Autodesk Fusion 360 part; units mm, degrees
(part 2 of 2)
sketch "Skizze5" plane through (0, 0, 6) normal (0, 0, 1) x (1, 0, 0)
  line L0 (-42, 58.3839) -> (-42, -1.6351) construction
  line L1 (-53.2037, 40.24) -> (-25.198, 40.24) construction
  line L2 (-52.8872, 9.76) -> (-24.0904, 9.76) construction
  line L3 (-69.9754, 25) -> (-16.6539, 25) construction
  line L4 (-40.2968, 37.29) -> (-38.5936, 40.24)
  line L5 (-38.5936, 40.24) -> (-40.2968, 43.19)
  line L6 (-40.2968, 43.19) -> (-43.7032, 43.19)
  line L7 (-43.7032, 43.19) -> (-45.4064, 40.24)
  line L8 (-45.4064, 40.24) -> (-43.7032, 37.29)
  line L9 (-43.7032, 37.29) -> (-40.2968, 37.29)
  line L10 (-40.2968, 6.81) -> (-38.5936, 9.76)
  line L11 (-38.5936, 9.76) -> (-40.2968, 12.71)
  line L12 (-40.2968, 12.71) -> (-43.7032, 12.71)
  line L13 (-43.7032, 12.71) -> (-45.4064, 9.76)
  line L14 (-45.4064, 9.76) -> (-43.7032, 6.81)
  line L15 (-43.7032, 6.81) -> (-40.2968, 6.81)
  line L16 (-28, 68.4623) -> (-28, -7.051) construction
  line L17 (-20.4, 58.9387) -> (-20.4, 26.026) construction
  line L18 (7.5, 60.7966) -> (7.5, 32.5289) construction
  line L19 (-25.5, 3.9958) -> (-25.5, -8.4792) construction
  line L20 (22.7, 6.3547) -> (22.7, -11) construction
  line L21 (16.5548, -1.7) -> (36, -1.7) construction
  line L22 (-31, 49.1) -> (26, 49.1) construction
  line L23 (-35.2993, -3) -> (-15, -3) construction
  point P0 (-42, 40.24)
  point P1 (-42, 9.76)
  point P2 (-42, 40.24)
  point P3 (-42, 9.76)
  point P4 (-25.5, -3)
  point P5 (22.7, -1.7)
  point P6 (-20.4, 49.1)
  dimension "d197" = 42
  dimension "d198" = 25
  dimension "d199" = 15.24
  dimension "d200" = 15.24
  dimension "d201" = 5.9
  dimension "d202" = 5.9
  dimension "d343" = 28
  dimension "d344" = 7.6
  dimension "d345" = 27.9
  dimension "d346" = 2.5
  dimension "d347" = 48.2
  dimension "d349" = 49.1
  dimension "d350" = 50.8
  dimension "d351" = 1.3
  constraint vertical L0
  constraint horizontal L1
  constraint horizontal L2
  constraint horizontal L3
  constraint coincident L1 P2
  constraint coincident L0 P2
  constraint coincident L2 P3
  constraint coincident L0 P3
  constraint coincident P2 P0
  constraint coincident P3 P1
  constraint vertical L16
  constraint perpendicular L3 L17
  constraint vertical L18
  constraint vertical L19
  constraint perpendicular L1 L20
  constraint perpendicular L20 L21
  constraint perpendicular L16 L22
  constraint perpendicular L16 L23
  constraint coincident L23 P4
  constraint coincident L19 P4
  constraint coincident L21 P5
  constraint coincident L20 P5
  constraint coincident L17 P6
  constraint coincident L22 P6
  measures "d197" distance of L0 origin
  measures "d198" distance of L3 origin
  measures "d199" distance of L1 L3
  measures "d200" distance of L2 L3
  measures "d201" distance of L6 L9
  measures "d202" distance of L12 L15
  measures "d343" distance of origin L16
  measures "d344" distance of L16 L17
  measures "d345" distance of L17 L18
  measures "d346" distance of L16 L19
  measures "d347" distance of L19 L20
  measures "d349" distance of origin L22
  measures "d350" distance of L21 L22
  measures "d351" distance of L21 L23
extrude "Extrusion12" cut sketch "Skizze5" along normal blind 2.6 bodies 11
sketch "Skizze6" plane through (0, 0, 10.3) normal (0, 0, 1) x (-1, 0, 0)
  circle A0 centre (42, -9.76) radius 4
  line L0 (93.3037, -25) -> (4.6405, -25) construction
  line L1 (42, -47.4403) -> (42, 6.0922) construction
  line L2 (54.3254, -40.24) -> (21.704, -40.24) construction
  line L3 (59.0095, -9.76) -> (18.86, -9.76) construction
  line L4 (33, -49.1) -> (-20.9546, -49.1) construction
  line L5 (33, 3) -> (13, 3) construction
  line L6 (-12.3565, 1.7) -> (-33, 1.7) construction
  line L7 (28, -59.161) -> (28, -2) construction
  line L8 (20.4, -59) -> (20.4, -30.5278) construction
  line L9 (25.5, -4.5907) -> (25.5, 13) construction
  line L10 (-22.7, -6.3058) -> (-22.7, 11) construction
  line L11 (-7.5, -59) -> (-7.5, -40) construction
  point P0 (42, -40.24)
  point P1 (42, -9.76)
  point P2 (20.4, -49.1)
  point P3 (25.5, 3)
  point P4 (20.4, -49.1)
  point P5 (-22.7, 1.7)
  dimension "d205" = 25
  dimension "d206" = 42
  dimension "d207" = 15.24
  dimension "d208" = 15.24
  dimension "d352" = 49.1
  dimension "d353" = 50.8
  dimension "d354" = 1.3
  dimension "d355" = 28
  dimension "d356" = 7.6
  dimension "d357" = 2.5
  dimension "d358" = 48.2
  dimension "d359" = 27.9
  constraint horizontal L0
  constraint vertical L1
  constraint horizontal L2
  constraint horizontal L3
  constraint coincident L2 P0
  constraint coincident L1 P0
  constraint coincident A0.centre P1
  constraint horizontal L4
  constraint horizontal L5
  constraint horizontal L6
  constraint perpendicular L4 L7
  constraint vertical L8
  constraint vertical L9
  constraint parallel L1 L10
  constraint vertical L11
  constraint coincident L5 P3
  constraint coincident L9 P3
  constraint coincident P4 P2
  constraint coincident L10 P5
  constraint coincident L6 P5
  measures "d205" distance of L0 origin
  measures "d206" distance of origin L1
  measures "d207" distance of L0 L2
  measures "d208" distance of L0 L3
  measures "d352" distance of L4 origin
  measures "d353" distance of L4 L6
  measures "d354" distance of L5 L6
  measures "d355" distance of origin L7
  measures "d356" distance of L7 L8
  measures "d357" distance of L7 L9
  measures "d358" distance of L9 L10
  measures "d359" distance of L11 P4
hole "Bohrung6" at (-42, 40.24, 10.3) at (-42, 9.76, 10.3) direction (0, 0, -1) diameter 3.5 depth 8.5 tip angle 180 bodies 11
extrude "Extrusion13" add sketch "Skizze1" along normal blind 2 separate body contours A41 makes body 27
extrude "Extrusion14" add sketch "Skizze1" along normal blind 3 contours A43 A50 | A43 A50 bodies 11
extrude "Extrusion15" add sketch "Skizze1" along normal blind 22.9 separate body contours L69 A55 | L36 L69 L95 A55 A56 makes body 28
extrude "Extrusion23" add sketch "Skizze1" along normal blind 10.3 contours L36 L69 L99 L103 A52 A53 | L69 L103 A52 | A57 L106 | A58 picked at (-22.0084, 48.4127) picked at (22.7471, -2.8734) bodies 11
sketch "Skizze7" plane through (0, 0, 22.9) normal (0, 0, 1) x (-1, 0, 0)
  arc A0 (-4.3775, -51.6) -> (-10.6225, -51.6) centre (-7.5, -49.1) ccw
  line L0 (-10.6225, -51.6) -> (-4.3775, -51.6)
  line L1 (20.4, -59.2047) -> (20.4, -39) construction
  line L2 (28, -63.0503) -> (28, 11) construction
  line L3 (25.5, -8) -> (25.5, 11) construction
  line L4 (-7.5, -58) -> (-7.5, -40) construction
  line L5 (-22.7, -5) -> (-22.7, 13) construction
  line L6 (33, -49.1) -> (-18.5705, -49.1) construction
  line L7 (-16.5833, 1.7) -> (-30, 1.7) construction
  line L8 (34, 3) -> (-38, 3) construction
  point P0 (20.4, -49.1024)
  point P1 (-7.5, -49.1)
  point P2 (-22.7, 1.7)
  point P3 (25.5, 3)
  dimension "d251" = 28
  dimension "d252" = 7.6
  dimension "d253" = 2.5
  dimension "d254" = 27.9
  dimension "d255" = 48.2
  dimension "d257" = 49.1
  dimension "d258" = 50.8
  dimension "d259" = 1.3
  constraint vertical L1
  constraint vertical L2
  constraint vertical L3
  constraint vertical L4
  constraint parallel L2 L5
  constraint perpendicular L4 L6
  constraint horizontal L7
  constraint perpendicular L2 L8
  constraint midpoint L1 P0
  constraint coincident P1 A0.centre
  constraint coincident L5 P2
  constraint coincident L7 P2
  constraint coincident L8 P3
  constraint coincident L3 P3
  measures "d251" distance of origin L2
  measures "d252" distance of L1 L2
  measures "d253" distance of L2 L3
  measures "d254" distance of L1 L4
  measures "d255" distance of L3 L5
  measures "d257" distance of origin L6
  measures "d258" distance of L6 L7
  measures "d259" distance of L7 L8
hole "Bohrung7" at (7.5, 49.1, 22.9) direction (0, 0, -1) diameter 2.4 depth 20 tip angle 180 bodies 11 28
hole "Bohrung11" at (-20.4, 49.1, 10.3) at (-25.5, -3, 10.3) at (22.7, -1.7, 10.3) direction (0, 0, -1) diameter 2.4 depth 8 tip angle 180 bodies 11
ref_plane "Arbeitsebene3" through (0, 0, 18.5) normal (0, 0, 1) x (1, 0, 0)
sketch "Skizze8" plane through (0, 0, 18.5) normal (0, 0, 1) x (1, 0, 0)
  line L0 (-32.3311, 49.1) -> (45.7753, 49.1) construction
  line L1 (-28, 60.5778) -> (-28, -21.6222) construction
  line L2 (-20.4, 58.6621) -> (-20.4, 30) construction
  line L3 (-28, 63.0503) -> (-28, -11)
  line L4 (7.5, 63.5287) -> (7.5, 26.5429) construction
  line L5 (-20.4, 59.2047) -> (-20.4, 39)
  line L6 (13.4256, -1.7) -> (50, -1.7) construction
  line L7 (22.7, 8.4795) -> (22.7, -22.342) construction
  line L8 (-25.5, 8) -> (-25.5, -11)
  line L9 (-35.5643, -3) -> (58.6845, -3) construction
  line L10 (-19.1298, 46.9024) -> (-17.8597, 49.1024)
  line L11 (-17.8597, 49.1024) -> (-19.1298, 51.3024)
  line L12 (-19.1298, 51.3024) -> (-21.6702, 51.3024)
  line L13 (-21.6702, 51.3024) -> (-22.9403, 49.1024)
  line L14 (-22.9403, 49.1024) -> (-21.6702, 46.9024)
  line L15 (-21.6702, 46.9024) -> (-19.1298, 46.9024)
  line L16 (8.7702, 46.9) -> (10.0403, 49.1)
  line L17 (10.0403, 49.1) -> (8.7702, 51.3)
  line L18 (8.7702, 51.3) -> (6.2298, 51.3)
  line L19 (6.2298, 51.3) -> (4.9597, 49.1)
  line L20 (4.9597, 49.1) -> (6.2298, 46.9)
  line L21 (6.2298, 46.9) -> (8.7702, 46.9)
  line L22 (23.9702, -3.9) -> (25.2403, -1.7)
  line L23 (25.2403, -1.7) -> (23.9702, 0.5)
  line L24 (23.9702, 0.5) -> (21.4298, 0.5)
  line L25 (21.4298, 0.5) -> (20.1597, -1.7)
  line L26 (20.1597, -1.7) -> (21.4298, -3.9)
  line L27 (21.4298, -3.9) -> (23.9702, -3.9)
  line L28 (-24.2298, -5.2) -> (-22.9597, -3)
  line L29 (-22.9597, -3) -> (-24.2298, -0.8)
  line L30 (-24.2298, -0.8) -> (-26.7702, -0.8)
  line L31 (-26.7702, -0.8) -> (-28.0403, -3)
  line L32 (-28.0403, -3) -> (-26.7702, -5.2)
  line L33 (-26.7702, -5.2) -> (-24.2298, -5.2)
  point P0 (22.7, -1.7)
  point P1 (-25.5, -3)
  point P2 (-20.4, 49.1024)
  point P3 (7.5, 49.1)
  point P4 (-20.4, 49.1024)
  point P5 (7.5, 49.1)
  point P6 (22.7, -1.7)
  point P7 (-25.5, -3)
  dimension "d264" = 49.1
  dimension "d265" = 28
  dimension "d266" = 7.6
  dimension "d267" = 27.9
  dimension "d268" = 50.8
  dimension "d269" = 48.2
  dimension "d270" = 1.3
  dimension "d271" = 4.4
  dimension "d272" = 4.4
  dimension "d273" = 4.4
  dimension "d274" = 4.4
  constraint horizontal L0
  constraint vertical L1
  constraint vertical L2
  constraint vertical L4
  constraint horizontal L6
  constraint parallel L4 L7
  constraint perpendicular L8 L9
  constraint coincident L6 P6
  constraint coincident L7 P6
  constraint coincident L9 P7
  constraint coincident L8 P7
  constraint midpoint L5 P4
  constraint coincident L4 P5
  constraint coincident L0 P5
  constraint coincident P4 P2
  constraint coincident P5 P3
  constraint coincident P6 P0
  constraint coincident P7 P1
  measures "d264" distance of L0 origin
  measures "d265" distance of origin L1
  measures "d266" distance of L2 L3
  measures "d267" distance of L4 L5
  measures "d268" distance of L0 L6
  measures "d269" distance of L7 L8
  measures "d270" distance of L6 L9
  measures "d271" distance of L12 L15
  measures "d272" distance of L18 L21
  measures "d273" distance of L24 L27
  measures "d274" distance of L30 L33
extrude "Extrusion16" cut sketch "Skizze8" along normal blind 1.9 contours L16 L17 L18 L19 L20 L21 bodies 28
ref_plane "Arbeitsebene5" through (0, 0, 6.7) normal (0, 0, 1) x (1, 0, 0)
sketch "Skizze12" plane through (0, 0, 6.7) normal (0, 0, 1) x (1, 0, 0)
  line L0 (-28, 61) -> (-28, -9) construction
  line L1 (-20.4, 58) -> (-20.4, 40) construction
  line L2 (-25.5, 3) -> (-25.5, -12) construction
  line L3 (22.7, 6) -> (22.7, -11) construction
  line L4 (-34, 49.1) -> (27, 49.1) construction
  line L5 (6, -1.7) -> (32.3027, -1.7) construction
  line L6 (-35, -3) -> (-10, -3) construction
  line L7 (-24.2298, -5.2) -> (-22.9597, -3)
  line L8 (-22.9597, -3) -> (-24.2298, -0.8)
  line L9 (-24.2298, -0.8) -> (-26.7702, -0.8)
  line L10 (-26.7702, -0.8) -> (-28.0403, -3)
  line L11 (-28.0403, -3) -> (-26.7702, -5.2)
  line L12 (-26.7702, -5.2) -> (-24.2298, -5.2)
  line L13 (23.9702, -3.9) -> (25.2403, -1.7)
  line L14 (25.2403, -1.7) -> (23.9702, 0.5)
  line L15 (23.9702, 0.5) -> (21.4298, 0.5)
  line L16 (21.4298, 0.5) -> (20.1597, -1.7)
  line L17 (20.1597, -1.7) -> (21.4298, -3.9)
  line L18 (21.4298, -3.9) -> (23.9702, -3.9)
  line L19 (-19.1298, 46.8) -> (-17.8597, 49)
  line L20 (-17.8597, 49) -> (-19.1298, 51.2)
  line L21 (-19.1298, 51.2) -> (-21.6702, 51.2)
  line L22 (-21.6702, 51.2) -> (-22.9403, 49)
  line L23 (-22.9403, 49) -> (-21.6702, 46.8)
  line L24 (-21.6702, 46.8) -> (-19.1298, 46.8)
  point P0 (22.7, -1.7)
  point P1 (-25.5, -3)
  point P2 (-20.4, 49)
  point P3 (-25.5, -3)
  point P4 (22.7, -1.7)
  point P5 (-20.4, 49)
  dimension "d364" = 28
  dimension "d365" = 7.6
  dimension "d366" = 2.5
  dimension "d367" = 48.2
  dimension "d368" = 49.1
  dimension "d369" = 50.8
  dimension "d370" = 1.3
  dimension "d371" = 4.4
  dimension "d372" = 4.4
  dimension "d373" = 4.4
  constraint vertical L0
  constraint parallel L0 L1
  constraint parallel L0 L2
  constraint parallel L1 L3
  constraint perpendicular L0 L4
  constraint perpendicular L0 L5
  constraint perpendicular L0 L6
  constraint coincident L3 P4
  constraint coincident L5 P4
  constraint coincident L2 P3
  constraint coincident L6 P3
  constraint midpoint L1 P5
  constraint coincident P3 P1
  constraint coincident P4 P0
  constraint coincident P5 P2
  measures "d364" distance of L0 origin
  measures "d365" distance of L0 L1
  measures "d366" distance of L0 L2
  measures "d367" distance of L2 L3
  measures "d368" distance of L4 origin
  measures "d369" distance of L4 L5
  measures "d370" distance of L5 L6
  measures "d371" distance of L15 L18
  measures "d372" distance of L9 L12
  measures "d373" distance of L21 L24
extrude "Extrusion20" add sketch "Skizze1" along normal blind 54 separate body contours L107 L108 L109 L110 L111 L112 A60 | A62 L117 L118 L119 L120 L121 L122 | A66 L129 L130 L131 L132 L133 L134 | A64 L123 L124 L125 L126 L127 L128 | A3 | A4 | A5 | A6 | A7 | A8 | A9 | A10 makes body 29 at (-78.8587, -52.2821, 36) makes body 30 at (-81.7969, 49.6043, 36) makes body 31 at (83.3987, -45.9658, 36) makes body 32 at (78.4698, 52.4983, 36)
ref_plane "Arbeitsebene4" through (0, 0, 45.9) normal (0, 0, 1) x (1, 0, 0)
sketch "Skizze10" plane through (0, 0, 45.9) normal (0, 0, 1) x (1, 0, 0)
  line L0 (76.3, 70) -> (76.3, -62.6845) construction
  line L1 (-76.3, 67.0452) -> (-76.3, -66.173) construction
  line L2 (-101.3259, 46.3) -> (105, 46.3) construction
  line L3 (-100, -46.3) -> (100, -46.3) construction
  line L4 (78.0032, 43.35) -> (79.7064, 46.3)
  line L5 (79.7064, 46.3) -> (78.0032, 49.25)
  line L6 (78.0032, 49.25) -> (74.5968, 49.25)
  line L7 (74.5968, 49.25) -> (72.8936, 46.3)
  line L8 (72.8936, 46.3) -> (74.5968, 43.35)
  line L9 (74.5968, 43.35) -> (78.0032, 43.35)
  line L10 (78.0032, -49.25) -> (79.7064, -46.3)
  line L11 (79.7064, -46.3) -> (78.0032, -43.35)
  line L12 (78.0032, -43.35) -> (74.5968, -43.35)
  line L13 (74.5968, -43.35) -> (72.8936, -46.3)
  line L14 (72.8936, -46.3) -> (74.5968, -49.25)
  line L15 (74.5968, -49.25) -> (78.0032, -49.25)
  line L16 (-74.5968, 43.35) -> (-72.8936, 46.3)
  line L17 (-72.8936, 46.3) -> (-74.5968, 49.25)
  line L18 (-74.5968, 49.25) -> (-78.0032, 49.25)
  line L19 (-78.0032, 49.25) -> (-79.7064, 46.3)
  line L20 (-79.7064, 46.3) -> (-78.0032, 43.35)
  line L21 (-78.0032, 43.35) -> (-74.5968, 43.35)
  line L22 (-74.5968, -49.25) -> (-72.8936, -46.3)
  line L23 (-72.8936, -46.3) -> (-74.5968, -43.35)
  line L24 (-74.5968, -43.35) -> (-78.0032, -43.35)
  line L25 (-78.0032, -43.35) -> (-79.7064, -46.3)
  line L26 (-79.7064, -46.3) -> (-78.0032, -49.25)
  line L27 (-78.0032, -49.25) -> (-74.5968, -49.25)
  point P0 (76.3, 46.3)
  point P1 (76.3, -46.3)
  point P2 (-76.3, 46.3)
  point P3 (-76.3, -46.3)
  dimension "d296" = 76.3
  dimension "d297" = 76.3
  dimension "d298" = 46.3
  dimension "d299" = 46.3
  dimension "d300" = 5.9
  dimension "d301" = 5.9
  dimension "d302" = 5.9
  dimension "d303" = 5.9
  constraint vertical L0
  constraint vertical L1
  constraint perpendicular L0 L2
  constraint horizontal L3
  constraint coincident L2 P0
  constraint coincident L0 P0
  constraint coincident L3 P1
  constraint coincident L0 P1
  constraint coincident L2 P2
  constraint coincident L1 P2
  constraint coincident L3 P3
  constraint coincident L1 P3
  measures "d296" distance of origin L0
  measures "d297" distance of origin L1
  measures "d298" distance of origin L2
  measures "d299" distance of origin L3
  measures "d300" distance of L6 L9
  measures "d301" distance of L18 L21
  measures "d302" distance of L24 L27
  measures "d303" distance of L12 L15
extrude "Extrusion24" cut sketch "Skizze12" along normal blind 1.9 bodies 11
sketch "Skizze11" plane through (0, 0, 54) normal (0, 0, 1) x (-1, 0, 0)
  line L0 (-71, -51.4) -> (-71, -41)
  line L1 (-71, -41) -> (-81.4, -41)
  line L2 (-81.4, -41) -> (-81.4, -44.2)
  line L3 (-81.4, -44.2) -> (-83.6, -44.2)
  arc A0 (-83.6, -44.2) -> (-74.2, -53.6) centre (-74, -44) ccw
  line L4 (-74.2, -53.6) -> (-74.2, -51.4)
  line L5 (-74.2, -51.4) -> (-71, -51.4)
  line L6 (-76.3, -49.5552) -> (-76.3, -32.6318) construction
  line L7 (-70.8, -40.8) -> (-70.8, -53.8)
  line L8 (-69, -46.3) -> (-87, -46.3) construction
  line L9 (-83.8, -40.8) -> (-70.8, -40.8)
  circle A1 centre (-76.3, -46.3) radius 3
  circle A2 centre (-76.3, -46.3) radius 4.65
  line L10 (0, -76.9494) -> (0, 87.0648) construction
  line L11 (107.4107, 0) -> (-122.5937, 0) construction
  circle A3 centre (76.3, -46.3) radius 3
  circle A4 centre (76.3, -46.3) radius 4.65
  circle A5 centre (76.3, 46.3) radius 4.65
  circle A6 centre (76.3, 46.3) radius 3
  circle A7 centre (-76.3, 46.3) radius 4.65
  circle A8 centre (-76.3, 46.3) radius 3
  point P0 (-76.3, -46.3)
  point P1 (-76.3, -46.3)
  point P2 (-76.3, 46.3)
  dimension "d322" = 5.5
  dimension "d323" = 5.5
  dimension "d324" = 6
  dimension "d325" = 9.3
  constraint vertical L6
  constraint horizontal L8
  constraint coincident L8 P1
  constraint coincident L6 P1
  constraint coincident P1 P0
  constraint vertical L10
  constraint horizontal L11
  constraint coincident L11 origin
  constraint coincident L10 origin
  constraint symmetric A1 L10 A3
  constraint symmetric A2 L10 A4
  constraint symmetric P1 L11 P2
  constraint symmetric A1 L11 A8
  constraint symmetric A2 L11 A7
  constraint symmetric L11 A3 A6
  constraint symmetric L11 A4 A5
  measures "d322" distance of L6 L7
  measures "d323" distance of L8 L9
  measures "d324" diameter of A1
  measures "d325" diameter of A2
hole "Bohrung10" at (76.3, 46.3, 54) at (-76.3, 46.3, 54) at (-76.3, -46.3, 54) at (76.3, -46.3, 54) direction (0, 0, -1) diameter 3.5 depth 15 tip angle 180 bodies 29 30 31 32
extrude "Extrusion21" cut sketch "Skizze11" against normal blind 3.5 contours A1 | A2 | A3 | A4 | A5 | A6 | A7 | A8 bodies 29 30 31 32
extrude "Extrusion22" cut sketch "Skizze10" along normal blind 2.6 bodies 29 30 31 32
